Autodesk Inventor part; units mm, degrees
(part 2 of 2)
  spline S97 degree 2 poles (210.6786, 189.7211) (210.6786, 190.1373) (210.1931, 190.6344) (209.8, 190.6344) knots 0 0 0 1 2 2 2
  line L388 (207.8954, 162.25) -> (207.8954, 163.1286)
  line L389 (207.8954, 163.1286) -> (209.589, 169.25)
  line L390 (209.589, 169.25) -> (210.826, 169.25)
  line L391 (210.826, 169.25) -> (209.1555, 163.354)
  line L392 (209.1555, 163.354) -> (210.6526, 163.354)
  line L393 (210.6526, 163.354) -> (210.6526, 164.3829)
  line L394 (210.6526, 164.3829) -> (211.8029, 164.3829)
  line L395 (211.8029, 164.3829) -> (211.8029, 162.25)
  line L396 (211.8029, 162.25) -> (207.8954, 162.25)
  spline S98 degree 2 poles (209.8087, 118.2905) (210.6237, 118.2905) (211.7104, 117.2789) (211.8087, 116.3656) knots 0 0 0 1 2 2 2
  line L397 (211.8087, 116.3656) -> (211.8087, 116.354)
  line L398 (211.8087, 116.354) -> (210.6584, 116.354)
  line L399 (210.6584, 116.354) -> (210.6584, 116.3598)
  spline S99 degree 2 poles (210.6584, 116.3598) (210.6179, 116.7471) (210.1613, 117.1806) (209.7971, 117.1806) knots 0 0 0 1 2 2 2
  spline S100 degree 2 poles (209.7971, 117.1806) (209.3867, 117.1806) (208.9416, 116.6315) (208.9416, 116.1402) knots 0 0 0 1 2 2 2
  line L400 (208.9416, 116.1402) -> (208.9416, 115.5506)
  spline S101 degree 2 poles (208.9416, 115.5506) (208.9416, 115.0535) (209.3636, 114.5159) (209.7624, 114.5159) knots 0 0 0 1 2 2 2
  spline S102 degree 2 poles (209.7624, 114.5159) (210.0283, 114.5159) (210.4618, 114.8049) (210.5948, 115.0708) knots 0 0 0 1 2 2 2
  line L401 (210.5948, 115.0708) -> (211.6584, 115.0708)
  line L402 (211.6584, 115.0708) -> (211.6584, 111.2095)
  line L403 (211.6584, 111.2095) -> (207.9936, 111.2095)
  line L404 (207.9936, 111.2095) -> (207.9936, 112.3136)
  line L405 (207.9936, 112.3136) -> (210.5081, 112.3136)
  line L406 (210.5081, 112.3136) -> (210.5081, 113.7182)
  spline S103 degree 2 poles (210.5081, 113.7182) (210.3347, 113.5679) (209.8491, 113.4061) (209.6121, 113.4061) knots 0 0 0 1 2 2 2
  spline S104 degree 2 poles (209.6121, 113.4061) (208.7451, 113.4061) (207.7913, 114.5275) (207.7913, 115.5506) knots 0 0 0 1 2 2 2
  line L407 (207.7913, 115.5506) -> (207.7913, 116.1402)
  spline S105 degree 2 poles (207.7913, 116.1402) (207.7913, 117.1691) (208.8491, 118.2905) (209.8087, 118.2905) knots 0 0 0 1 2 2 2
  line L408 (212.3467, 92.0147) -> (212.3467, 90.8322)
  line L409 (212.3467, 90.8322) -> (209.7703, 85.25)
  line L410 (209.7703, 85.25) -> (208.3434, 85.25)
  line L411 (208.3434, 85.25) -> (210.8471, 90.7661)
  line L412 (210.8471, 90.7661) -> (207.0948, 90.7661)
  line L413 (207.0948, 90.7661) -> (207.0948, 92.0147)
  line L414 (207.0948, 92.0147) -> (212.3467, 92.0147)
  line L415 (209.004, 93.25) -> (209.004, 88.5398)
  line L416 (209.004, 88.5398) -> (207.7026, 88.5398)
  line L417 (207.7026, 88.5398) -> (207.7026, 93.25)
  line L418 (207.7026, 93.25) -> (209.004, 93.25)
  spline S106 degree 2 poles (209.852, 67.3309) (210.459, 67.3309) (211.4012, 66.8801) (211.9618, 66.0361) (212.0197, 65.435) knots 0 0 0 1 2 3 3 3
  line L419 (212.0197, 65.435) -> (210.8347, 65.435)
  spline S107 degree 2 poles (210.8347, 65.435) (210.7769, 65.828) (210.2971, 66.2211) (209.9214, 66.2211) knots 0 0 0 1 2 2 2
  spline S108 degree 2 poles (209.9214, 66.2211) (209.4879, 66.2211) (209.0197, 65.7471) (209.0197, 65.3194) knots 0 0 0 1 2 2 2
  line L420 (209.0197, 65.3194) -> (209.0197, 65.1286)
  spline S109 degree 2 poles (209.0197, 65.1286) (209.0197, 64.6662) (209.4358, 64.1575) (209.8231, 64.1575) knots 0 0 0 1 2 2 2
  line L421 (209.8231, 64.1575) -> (210.3723, 64.1575)
  line L422 (210.3723, 64.1575) -> (210.3723, 63.0535)
  line L423 (210.3723, 63.0535) -> (209.8231, 63.0535)
  spline S110 degree 2 poles (209.8231, 63.0535) (209.4936, 63.0535) (209.1353, 62.6199) (209.1353, 62.2211) knots 0 0 0 1 2 2 2
  line L424 (209.1353, 62.2211) -> (209.1353, 62.0535)
  spline S111 degree 2 poles (209.1353, 62.0535) (209.1353, 61.6777) (209.5225, 61.2789) (209.8809, 61.2789) knots 0 0 0 1 2 2 2
  spline S112 degree 2 poles (209.8809, 61.2789) (210.1988, 61.2789) (210.6439, 61.6893) (210.7249, 62.1055) knots 0 0 0 1 2 2 2
  line L425 (210.7249, 62.1055) -> (211.904, 62.1055)
  spline S113 degree 2 poles (211.904, 62.1055) (211.7884, 61.1806) (210.6786, 60.1691) (209.852, 60.1691) knots 0 0 0 1 2 2 2
  spline S114 degree 2 poles (209.852, 60.1691) (208.9329, 60.1691) (207.9329, 61.1171) (207.9329, 61.9899) knots 0 0 0 1 2 2 2
  line L426 (207.9329, 61.9899) -> (207.9329, 62.1575)
  spline S115 degree 2 poles (207.9329, 62.1575) (207.9329, 62.6604) (208.4647, 63.4118) (208.9503, 63.591) knots 0 0 0 1 2 2 2
  spline S116 degree 2 poles (208.9503, 63.591) (208.4127, 63.7066) (207.8173, 64.5679) (207.8173, 65.2327) knots 0 0 0 1 2 2 2
  line L427 (207.8173, 65.2327) -> (207.8173, 65.3945)
  spline S117 degree 2 poles (207.8173, 65.3945) (207.8173, 66.3194) (208.8809, 67.3309) (209.852, 67.3309) knots 0 0 0 1 2 2 2
  line L428 (211.7827, 41.7905) -> (211.7827, 40.7673)
  line L429 (211.7827, 40.7673) -> (209.3607, 37.5592)
  spline S118 degree 2 poles (209.3607, 37.5592) (209.1699, 37.3107) (208.9618, 36.7847) (208.9618, 36.5592) knots 0 0 0 1 2 2 2
  line L430 (208.9618, 36.5592) -> (208.9618, 36.5535)
  spline S119 degree 2 poles (208.9618, 36.5535) (208.9618, 36.2009) (209.3954, 35.8136) (209.7884, 35.8136) knots 0 0 0 1 2 2 2
  spline S120 degree 2 poles (209.7884, 35.8136) (210.1584, 35.8136) (210.6324, 36.2818) (210.6844, 36.7095) knots 0 0 0 1 2 2 2
  line L431 (210.6844, 36.7095) -> (210.6844, 36.7153)
  line L432 (210.6844, 36.7153) -> (211.8694, 36.7153)
  line L433 (211.8694, 36.7153) -> (211.8694, 36.7095)
  spline S121 degree 2 poles (211.8694, 36.7095) (211.7653, 35.7558) (210.6671, 34.7095) (209.7942, 34.7095) knots 0 0 0 1 2 2 2
  spline S122 degree 2 poles (209.7942, 34.7095) (208.8289, 34.7095) (207.7769, 35.6633) (207.7769, 36.5361) knots 0 0 0 1 2 2 2
  line L434 (207.7769, 36.5361) -> (207.7769, 36.5419)
  spline S123 degree 2 poles (207.7769, 36.5419) (207.7769, 36.9639) (208.0948, 37.8425) (208.3838, 38.2182) knots 0 0 0 1 2 2 2
  line L435 (208.3838, 38.2182) -> (210.2566, 40.6864)
  line L436 (210.2566, 40.6864) -> (207.7364, 40.6864)
  line L437 (207.7364, 40.6864) -> (207.7364, 41.7905)
  line L438 (207.7364, 41.7905) -> (211.7827, 41.7905)
  line L439 (208.9763, 9.25) -> (208.9763, 16.25)
  line L440 (208.9763, 16.25) -> (210.1266, 16.25)
  line L441 (210.1266, 16.25) -> (210.1266, 10.5564)
  line L442 (210.1266, 10.5564) -> (211.0514, 11.0246)
  line L443 (211.0514, 11.0246) -> (211.0514, 9.8165)
  line L444 (211.0514, 9.8165) -> (210.0341, 9.25)
  line L445 (210.0341, 9.25) -> (208.9763, 9.25)
  line L446 (192.4488, -8.8562) -> (192.4488, -2.7562)
  line L447 (192.4488, -2.7562) -> (193.4512, -2.7562)
  line L448 (193.4512, -2.7562) -> (193.4512, -8.8562)
  line L449 (193.4512, -8.8562) -> (192.4488, -8.8562)
  line L450 (189.0488, -8.8562) -> (189.0488, -2.7562)
  line L451 (189.0488, -2.7562) -> (190.0512, -2.7562)
  line L452 (190.0512, -2.7562) -> (190.0512, -8.8562)
  line L453 (190.0512, -8.8562) -> (189.0488, -8.8562)
  line L454 (189.5777, -6.3225) -> (189.5777, -5.3604)
  line L455 (189.5777, -5.3604) -> (193.0483, -5.3604)
  line L456 (193.0483, -5.3604) -> (193.0483, -6.3225)
  line L457 (193.0483, -6.3225) -> (189.5777, -6.3225)
  line L458 (165.823, -5.5003) -> (167.9386, -5.5003)
  line L459 (167.9386, -5.5003) -> (167.9386, -6.6286)
  spline S124 degree 2 poles (167.9386, -6.6286) (167.9386, -7.3187) (167.3946, -8.3463) (166.4225, -8.9155) (165.7626, -8.9155) knots 0 0 0 1 2 3 3 3
  spline S125 degree 2 poles (165.7626, -8.9155) (165.1027, -8.9155) (164.1104, -8.3815) (163.5614, -7.4144) (163.5614, -6.7646) knots 0 0 0 1 2 3 3 3
  line L460 (163.5614, -6.7646) -> (163.5614, -4.9663)
  spline S126 degree 2 poles (163.5614, -4.9663) (163.5614, -4.2763) (164.1054, -3.2537) (165.0826, -2.6845) (165.7374, -2.6845) knots 0 0 0 1 2 3 3 3
  spline S127 degree 2 poles (165.7374, -2.6845) (166.2764, -2.6845) (167.173, -3.1379) (167.7825, -3.9539) (167.8883, -4.4979) knots 0 0 0 1 2 3 3 3
  line L461 (167.8883, -4.4979) -> (166.8053, -4.4979)
  spline S128 degree 2 poles (166.8053, -4.4979) (166.7045, -4.11) (166.09, -3.697) (165.7374, -3.697) knots 0 0 0 1 2 2 2
  spline S129 degree 2 poles (165.7374, -3.697) (165.2186, -3.697) (164.594, -4.3921) (164.594, -4.9663) knots 0 0 0 1 2 2 2
  line L462 (164.594, -4.9663) -> (164.594, -6.7646)
  spline S130 degree 2 poles (164.594, -6.7646) (164.594, -7.2834) (165.2337, -7.903) (165.7626, -7.903) knots 0 0 0 1 2 2 2
  spline S131 degree 2 poles (165.7626, -7.903) (166.2814, -7.898) (166.906, -7.2381) (166.906, -6.6488) knots 0 0 0 1 2 2 2
  line L463 (166.906, -6.6488) -> (166.906, -6.4624)
  line L464 (166.906, -6.4624) -> (165.823, -6.4624)
  line L465 (165.823, -6.4624) -> (165.823, -5.5003)
  line L466 (138.5626, -8.85) -> (138.5626, -2.75)
  line L467 (138.5626, -2.75) -> (139.5649, -2.75)
  line L468 (139.5649, -2.75) -> (139.5649, -8.85)
  line L469 (139.5649, -8.85) -> (138.5626, -8.85)
  line L470 (138.9806, -3.7121) -> (138.9806, -2.75)
  line L471 (138.9806, -2.75) -> (142.4815, -2.75)
  line L472 (142.4815, -2.75) -> (142.4815, -3.7121)
  line L473 (142.4815, -3.7121) -> (138.9806, -3.7121)
  line L474 (138.9806, -6.3516) -> (138.9806, -5.3895)
  line L475 (138.9806, -5.3895) -> (142.0231, -5.3945)
  line L476 (142.0231, -5.3945) -> (142.0231, -6.3516)
  line L477 (142.0231, -6.3516) -> (138.9806, -6.3516)
  line L478 (112.8963, -8.85) -> (112.8963, -2.75)
  line L479 (112.8963, -2.75) -> (113.8987, -2.75)
  line L480 (113.8987, -2.75) -> (113.8987, -8.85)
  line L481 (113.8987, -8.85) -> (112.8963, -8.85)
  line L482 (113.3094, -3.7121) -> (113.3094, -2.75)
  line L483 (113.3094, -2.75) -> (116.8958, -2.75)
  line L484 (116.8958, -2.75) -> (116.8958, -3.7121)
  line L485 (116.8958, -3.7121) -> (113.3094, -3.7121)
  line L486 (113.3094, -8.85) -> (113.3094, -7.8879)
  line L487 (113.3094, -7.8879) -> (116.8958, -7.8879)
  line L488 (116.8958, -7.8879) -> (116.8958, -8.85)
  line L489 (116.8958, -8.85) -> (113.3094, -8.85)
  line L490 (113.3094, -6.3012) -> (113.3094, -5.3391)
  line L491 (113.3094, -5.3391) -> (116.4374, -5.3441)
  line L492 (116.4374, -5.3441) -> (116.4374, -6.3012)
  line L493 (116.4374, -6.3012) -> (113.3094, -6.3012)
  line L494 (87.7237, -8.85) -> (87.7237, -7.8879)
  line L495 (87.7237, -7.8879) -> (89.1442, -7.8879)
  spline S132 degree 2 poles (89.1442, -7.8879) (89.7638, -7.8879) (90.4488, -7.2633) (90.4488, -6.6991) knots 0 0 0 1 2 2 2
  line L496 (90.4488, -6.6991) -> (90.4488, -4.9009)
  spline S133 degree 2 poles (90.4488, -4.9009) (90.4488, -4.3317) (89.7638, -3.7121) (89.1442, -3.7121) knots 0 0 0 1 2 2 2
  line L497 (89.1442, -3.7121) -> (87.7237, -3.7121)
  line L498 (87.7237, -3.7121) -> (87.7237, -2.75)
  line L499 (87.7237, -2.75) -> (89.119, -2.75)
  spline S134 degree 2 poles (89.119, -2.75) (90.2474, -2.75) (91.4815, -3.8934) (91.4815, -4.9361) knots 0 0 0 1 2 2 2
  line L500 (91.4815, -4.9361) -> (91.4815, -6.6639)
  spline S135 degree 2 poles (91.4815, -6.6639) (91.4815, -7.3338) (90.9374, -8.3161) (89.8847, -8.85) (89.114, -8.85) knots 0 0 0 1 2 3 3 3
  line L501 (89.114, -8.85) -> (87.7237, -8.85)
  line L502 (87.1445, -8.85) -> (87.1445, -2.75)
  line L503 (87.1445, -2.75) -> (88.1469, -2.75)
  line L504 (88.1469, -2.75) -> (88.1469, -8.85)
  line L505 (88.1469, -8.85) -> (87.1445, -8.85)
  spline S136 degree 2 poles (63.8407, -8.9155) (63.1758, -8.9155) (62.2036, -8.3664) (61.6797, -7.3389) (61.6797, -6.6387) knots 0 0 0 1 2 3 3 3
  line L506 (61.6797, -6.6387) -> (61.6797, -4.9663)
  spline S137 degree 2 poles (61.6797, -4.9663) (61.6797, -4.2561) (62.2036, -3.2336) (63.1758, -2.6845) (63.8407, -2.6845) knots 0 0 0 1 2 3 3 3
  spline S138 degree 2 poles (63.8407, -2.6845) (64.3948, -2.6845) (65.2863, -3.158) (65.8757, -4.0345) (65.9865, -4.644) knots 0 0 0 1 2 3 3 3
  line L507 (65.9865, -4.644) -> (64.9539, -4.644)
  spline S139 degree 2 poles (64.9539, -4.644) (64.8783, -4.3417) (64.5509, -3.9136) (64.1026, -3.6768) (63.8407, -3.6768) knots 0 0 0 1 2 3 3 3
  spline S140 degree 2 poles (63.8407, -3.6768) (63.3218, -3.6768) (62.7123, -4.372) (62.7123, -4.9663) knots 0 0 0 1 2 2 2
  line L508 (62.7123, -4.9663) -> (62.7123, -6.6437)
  spline S141 degree 2 poles (62.7123, -6.6437) (62.7123, -7.2331) (63.3218, -7.9232) (63.8407, -7.9232) knots 0 0 0 1 2 2 2
  spline S142 degree 2 poles (63.8407, -7.9232) (64.2336, -7.9232) (64.8481, -7.4245) (64.9539, -6.956) knots 0 0 0 1 2 2 2
  line L509 (64.9539, -6.956) -> (65.9865, -6.956)
  spline S143 degree 2 poles (65.9865, -6.956) (65.8757, -7.5605) (65.2813, -8.442) (64.3948, -8.9155) (63.8407, -8.9155) knots 0 0 0 1 2 3 3 3
  point P0 (0, 0)
  point P1 (0.0104, 102.0099)
  point P2 (1.1, -1.1)
  point P3 (179.6, -1.1)
  point P4 (202.9, -10.5)
  point P5 (-1.1, 1.1)
  point P6 (-10.5, 24.4)
  point P7 (-1.1, 26.6)
  point P8 (-10.5, 49.9)
  point P9 (-1.1, 52.1)
  point P10 (-1.1, 77.6)
  point P11 (-1.1, 154.1)
  point P12 (1.1, 214.5)
  point P13 (24.4, 205.1)
  point P14 (26.6, 214.5)
  point P15 (52.1, 214.5)
  point P16 (214.5, 1.1)
  point P17 (205.1, 24.4)
  point P18 (214.5, 26.6)
  point P19 (205.1, 49.9)
  point P20 (205.1, 75.4)
  point P21 (214.5, 154.1)
  dimension "d0" = 25.5
  dimension "d1" = 25.5
  constraints: 100 coincident, 4 point on line, 2 horizontal, 1 vertical, 72 other
extrude "Extrusion10" cut sketch "Sketch10" against normal blind 0.3 contours S0 | S2 | L198 L199 L200 L201 L202 L208 L207 L206 L203 L205 L204 | L208 L205 L206 L203 | L203 L206 L202 L208 | L202 L206 L207 L208 | L223 L220 L221 L216 L215 L222 L214 L213 L212 L210 L209 | L209 L210 L222 L219 | L222 L210 S4 L211 S5 L212 L214 S6 S7 L215 L217 S8 S9 S10 L218 S11 L219 | L212 L213 L214 L222 | L217 L222 L215 L216 | S12 L224 S13 S14 L225 S15 S16 L226 S17 S18 L227 S19 | L232 L233 L234 L235 L236 L237 L238 L239 L240 | S28 L241 L242 L243 S29 S30 L244 S31 S32 L245 L246 L247 L248 L249 L250 S33 S34 L251 S35 | L252 L253 L254 L255 L256 L259 L258 | L259 L256 L261 L258 | L258 L261 L262 L259 | L261 L256 L257 L258 | L259 L260 L261 L256 | S36 L263 S37 S38 L264 S39 L265 L266 L267 S40 L268 S41 S42 L269 S43 S44 L270 S45 S46 L271 S47 | L272 L273 S48 L274 S49 S50 L275 L276 L277 S51 S52 L278 S53 L279 L280 L281 L282 | L283 L284 L285 L286 L287 L288 L289 | L290 L291 L292 L293 L294 L300 L299 L298 L295 L297 L296 | L300 L297 L298 L295 | L295 L298 L294 L300 | L294 L298 L299 L300 | L315 L312 L313 L308 L307 L314 L306 L305 L304 L302 L301 | L301 L302 L314 L311 | L314 L302 S54 L303 S55 L304 L306 S56 S57 L307 L309 S58 S59 S60 L310 S61 L311 | L304 L305 L306 L314 | L309 L314 L307 L308 | S62 L316 S63 S64 L317 S65 S66 L318 S67 S68 L319 S69 | L331 L328 L329 L324 L323 L330 L321 L320 | L320 L321 L330 L327 | L330 L321 S70 L322 S71 L323 L325 S72 L326 S73 L327 | L323 L324 L325 L330 | L332 L333 L336 L339 L334 L345 L344 L347 L341 L340 L335 | L340 L341 L334 L335 | L333 L334 L339 L336 | L334 L341 L342 L343 | L337 L338 L339 L334 | L347 L344 L345 L334 | L334 L345 L346 L347 | L348 L349 L352 L355 L350 L357 L356 L359 L351 | L349 L350 L355 L352 | L359 L356 L357 L350 | L350 L357 L358 L359 | L353 L354 L355 L350 | L360 L361 S74 S75 L362 S76 S77 L363 S78 S79 L364 S80 S81 L365 L366 L367 | L368 L369 L370 L377 L376 L379 L371 | L379 L376 L377 L370 | L370 L377 L372 L379 | L379 L378 L377 L372 L373 L374 L375 | L372 L377 L378 L379 | S82 L380 S83 S84 L381 S85 S86 L382 S87 S88 L383 S89 | L388 L389 L390 L391 L392 L393 L394 L395 L396 | S98 L397 L398 L399 S99 S100 L400 S101 S102 L401 L402 L403 L404 L405 L406 S103 S104 L407 S105 | L408 L409 L410 L411 L412 L415 L414 | L415 L412 L417 L414 | L414 L417 L418 L415 | L417 L412 L413 L414 | L415 L416 L417 L412 | S106 L419 S107 S108 L420 S109 L421 L422 L423 S110 L424 S111 S112 L425 S113 S114 L426 S115 S116 L427 S117 | L428 L429 S118 L430 S119 S120 L431 L432 L433 S121 S122 L434 S123 L435 L436 L437 L438 | L439 L440 L441 L442 L443 L444 L445 | L446 L457 L456 L455 L447 L448 L449 | L457 L452 L455 L446 | L446 L455 L456 L457 | L457 L454 L455 L452 | L452 L453 L450 L451 L455 L454 L457 | L458 L459 S124 S125 L460 S126 S127 L461 S128 S129 L462 S130 S131 L463 L464 L465 | L466 L467 L470 L473 L468 L475 L474 L477 L469 | L467 L468 L473 L470 | L477 L474 L475 L468 | L468 L475 L476 L477 | L471 L472 L473 L468 | L478 L479 L482 L485 L480 L491 L490 L493 L487 L486 L481 | L486 L487 L480 L481 | L479 L480 L485 L482 | L480 L487 L488 L489 | L483 L484 L485 L480 | L493 L490 L491 L480 | L480 L491 L492 L493 | L505 L502 L503 L498 L497 L504 L495 L494 | L494 L495 L504 L501 | L504 L495 S132 L496 S133 L497 L499 S134 L500 S135 L501 | L497 L498 L499 L504 | S136 L506 S137 S138 L507 S139 S140 L508 S141 S142 L509 S143
sketch "Sketch11" plane through (0, 2.8, 0) normal (0, 1, 0) x (1, 0, 0)
  circle A0 centre (12.75, 191.25) radius 3 projected
  circle A1 centre (38.25, 191.25) radius 3 projected
  circle A2 centre (63.75, 191.25) radius 3 projected
  circle A3 centre (89.25, 191.25) radius 3 projected
  circle A4 centre (114.75, 191.25) radius 3 projected
  circle A5 centre (140.25, 191.25) radius 3 projected
  circle A6 centre (165.75, 191.25) radius 3 projected
  circle A7 centre (191.25, 191.25) radius 3 projected
  circle A8 centre (191.25, 165.75) radius 3 projected
  circle A9 centre (165.75, 165.75) radius 3 projected
  circle A10 centre (114.75, 165.75) radius 3 projected
  circle A11 centre (63.75, 165.75) radius 3 projected
  circle A12 centre (89.25, 140.25) radius 3 projected
  circle A13 centre (89.25, 165.75) radius 3 projected
  circle A14 centre (38.25, 165.75) radius 3 projected
  circle A15 centre (12.75, 165.75) radius 3 projected
  circle A16 centre (140.25, 165.75) radius 3 projected
  circle A17 centre (191.25, 140.25) radius 3 projected
  circle A18 centre (165.75, 140.25) radius 3 projected
  circle A19 centre (140.25, 140.25) radius 3 projected
  circle A20 centre (114.75, 140.25) radius 3 projected
  circle A21 centre (114.75, 114.75) radius 3 projected
  circle A22 centre (165.75, 114.75) radius 3 projected
  circle A23 centre (140.25, 89.25) radius 3 projected
  circle A24 centre (140.25, 114.75) radius 3 projected
  circle A25 centre (191.25, 114.75) radius 3 projected
  circle A26 centre (89.25, 114.75) radius 3 projected
  circle A27 centre (63.75, 114.75) radius 3 projected
  circle A28 centre (38.25, 114.75) radius 3 projected
  circle A29 centre (12.75, 114.75) radius 3 projected
  circle A30 centre (38.25, 89.25) radius 3 projected
  circle A31 centre (12.75, 89.25) radius 3 projected
  circle A32 centre (63.75, 89.25) radius 3 projected
  circle A33 centre (89.25, 89.25) radius 3 projected
  circle A34 centre (63.75, 140.25) radius 3 projected
  circle A35 centre (38.25, 140.25) radius 3 projected
  circle A36 centre (12.75, 140.25) radius 3 projected
  circle A37 centre (114.75, 89.25) radius 3 projected
  circle A38 centre (165.75, 89.25) radius 3 projected
  circle A39 centre (191.25, 89.25) radius 3 projected
  circle A40 centre (191.25, 63.75) radius 3 projected
  circle A41 centre (165.75, 63.75) radius 3 projected
  circle A42 centre (89.25, 63.75) radius 3 projected
  circle A43 centre (140.25, 63.75) radius 3 projected
  circle A44 centre (114.75, 63.75) radius 3 projected
  circle A45 centre (63.75, 63.75) radius 3 projected
  circle A46 centre (38.25, 63.75) radius 3 projected
  circle A47 centre (12.75, 63.75) radius 3 projected
  circle A48 centre (191.25, 38.25) radius 3 projected
  circle A49 centre (165.75, 38.25) radius 3 projected
  circle A50 centre (140.25, 38.25) radius 3 projected
  circle A51 centre (114.75, 38.25) radius 3 projected
  circle A52 centre (89.25, 38.25) radius 3 projected
  circle A53 centre (63.75, 38.25) radius 3 projected
  circle A54 centre (38.25, 38.25) radius 3 projected
  circle A55 centre (12.75, 38.25) radius 3 projected
  circle A56 centre (12.75, 12.75) radius 3 projected
  circle A57 centre (38.25, 12.75) radius 3 projected
  circle A58 centre (63.75, 12.75) radius 3 projected
  circle A59 centre (89.25, 12.75) radius 3 projected
  circle A60 centre (114.75, 12.75) radius 3 projected
  circle A61 centre (140.25, 12.75) radius 3 projected
  circle A62 centre (165.75, 12.75) radius 3 projected
  circle A63 centre (191.25, 12.75) radius 3 projected
  circle A64 centre (5.5, 198.5) radius 1.75
  circle A65 centre (20, 184) radius 1.75
  line L0 (1.5, 202.5) -> (24, 202.5) projected
  line L1 (1.5, 180) -> (1.5, 202.5) projected
  line L2 (24, 180) -> (1.5, 180) projected
  line L3 (24, 202.5) -> (24, 180) projected
  circle A66 centre (31, 198.5) radius 1.75
  circle A67 centre (45.5, 184) radius 1.75
  circle A68 centre (56.5, 198.5) radius 1.75
  circle A69 centre (71, 184) radius 1.75
  circle A70 centre (82, 198.5) radius 1.75
  circle A71 centre (96.5, 184) radius 1.75
  circle A72 centre (107.5, 198.5) radius 1.75
  circle A73 centre (122, 184) radius 1.75
  circle A74 centre (133, 198.5) radius 1.75
  circle A75 centre (147.5, 184) radius 1.75
  circle A76 centre (158.5, 198.5) radius 1.75
  circle A77 centre (173, 184) radius 1.75
  circle A78 centre (184, 198.5) radius 1.75
  circle A79 centre (198.5, 184) radius 1.75
  circle A80 centre (5.5, 173) radius 1.75
  circle A81 centre (20, 158.5) radius 1.75
  circle A82 centre (31, 173) radius 1.75
  circle A83 centre (45.5, 158.5) radius 1.75
  circle A84 centre (56.5, 173) radius 1.75
  circle A85 centre (71, 158.5) radius 1.75
  circle A86 centre (82, 173) radius 1.75
  circle A87 centre (96.5, 158.5) radius 1.75
  circle A88 centre (107.5, 173) radius 1.75
  circle A89 centre (122, 158.5) radius 1.75
  circle A90 centre (133, 173) radius 1.75
  circle A91 centre (147.5, 158.5) radius 1.75
  circle A92 centre (158.5, 173) radius 1.75
  circle A93 centre (173, 158.5) radius 1.75
  circle A94 centre (184, 173) radius 1.75
  circle A95 centre (198.5, 158.5) radius 1.75
  circle A96 centre (5.5, 147.5) radius 1.75
  circle A97 centre (20, 133) radius 1.75
  circle A98 centre (31, 147.5) radius 1.75
  circle A99 centre (45.5, 133) radius 1.75
  circle A100 centre (56.5, 147.5) radius 1.75
  circle A101 centre (71, 133) radius 1.75
  circle A102 centre (82, 147.5) radius 1.75
  circle A103 centre (96.5, 133) radius 1.75
  circle A104 centre (107.5, 147.5) radius 1.75
  circle A105 centre (122, 133) radius 1.75
  circle A106 centre (133, 147.5) radius 1.75
  circle A107 centre (147.5, 133) radius 1.75
  circle A108 centre (158.5, 147.5) radius 1.75
  circle A109 centre (173, 133) radius 1.75
  circle A110 centre (184, 147.5) radius 1.75
  circle A111 centre (198.5, 133) radius 1.75
  circle A112 centre (5.5, 122) radius 1.75
  circle A113 centre (20, 107.5) radius 1.75
  circle A114 centre (31, 122) radius 1.75
  circle A115 centre (45.5, 107.5) radius 1.75
  circle A116 centre (56.5, 122) radius 1.75
  circle A117 centre (71, 107.5) radius 1.75
  circle A118 centre (82, 122) radius 1.75
  circle A119 centre (96.5, 107.5) radius 1.75
  circle A120 centre (107.5, 122) radius 1.75
  circle A121 centre (122, 107.5) radius 1.75
  circle A122 centre (133, 122) radius 1.75
  circle A123 centre (147.5, 107.5) radius 1.75
  circle A124 centre (158.5, 122) radius 1.75
  circle A125 centre (173, 107.5) radius 1.75
  circle A126 centre (184, 122) radius 1.75
  circle A127 centre (198.5, 107.5) radius 1.75
  circle A128 centre (5.5, 96.5) radius 1.75
  circle A129 centre (20, 82) radius 1.75
  circle A130 centre (31, 96.5) radius 1.75
  circle A131 centre (45.5, 82) radius 1.75
  circle A132 centre (56.5, 96.5) radius 1.75
  circle A133 centre (71, 82) radius 1.75
  circle A134 centre (82, 96.5) radius 1.75
  circle A135 centre (96.5, 82) radius 1.75
  circle A136 centre (107.5, 96.5) radius 1.75
  circle A137 centre (122, 82) radius 1.75
  circle A138 centre (133, 96.5) radius 1.75
  circle A139 centre (147.5, 82) radius 1.75
  circle A140 centre (158.5, 96.5) radius 1.75
  circle A141 centre (173, 82) radius 1.75
  circle A142 centre (184, 96.5) radius 1.75
  circle A143 centre (198.5, 82) radius 1.75
  circle A144 centre (5.5, 71) radius 1.75
  circle A145 centre (20, 56.5) radius 1.75
  circle A146 centre (31, 71) radius 1.75
  circle A147 centre (45.5, 56.5) radius 1.75
  circle A148 centre (56.5, 71) radius 1.75
  circle A149 centre (71, 56.5) radius 1.75
  circle A150 centre (82, 71) radius 1.75
  circle A151 centre (96.5, 56.5) radius 1.75
  circle A152 centre (107.5, 71) radius 1.75
  circle A153 centre (122, 56.5) radius 1.75
  circle A154 centre (133, 71) radius 1.75
  circle A155 centre (147.5, 56.5) radius 1.75
  circle A156 centre (158.5, 71) radius 1.75
  circle A157 centre (173, 56.5) radius 1.75
  circle A158 centre (184, 71) radius 1.75
  circle A159 centre (198.5, 56.5) radius 1.75
  circle A160 centre (5.5, 45.5) radius 1.75
  circle A161 centre (20, 31) radius 1.75
  circle A162 centre (31, 45.5) radius 1.75
  circle A163 centre (45.5, 31) radius 1.75
  circle A164 centre (56.5, 45.5) radius 1.75
  circle A165 centre (71, 31) radius 1.75
  circle A166 centre (82, 45.5) radius 1.75
  circle A167 centre (96.5, 31) radius 1.75
  circle A168 centre (107.5, 45.5) radius 1.75
  circle A169 centre (122, 31) radius 1.75
  circle A170 centre (133, 45.5) radius 1.75
  circle A171 centre (147.5, 31) radius 1.75
  circle A172 centre (158.5, 45.5) radius 1.75
  circle A173 centre (173, 31) radius 1.75
  circle A174 centre (184, 45.5) radius 1.75
  circle A175 centre (198.5, 31) radius 1.75
  circle A176 centre (5.5, 20) radius 1.75
  circle A177 centre (20, 5.5) radius 1.75
  circle A178 centre (31, 20) radius 1.75
  circle A179 centre (45.5, 5.5) radius 1.75
  circle A180 centre (56.5, 20) radius 1.75
  circle A181 centre (71, 5.5) radius 1.75
  circle A182 centre (82, 20) radius 1.75
  circle A183 centre (96.5, 5.5) radius 1.75
  circle A184 centre (107.5, 20) radius 1.75
  circle A185 centre (122, 5.5) radius 1.75
  circle A186 centre (133, 20) radius 1.75
  circle A187 centre (147.5, 5.5) radius 1.75
  circle A188 centre (158.5, 20) radius 1.75
  circle A189 centre (173, 5.5) radius 1.75
  circle A190 centre (184, 20) radius 1.75
  circle A191 centre (198.5, 5.5) radius 1.75
  line L4 (202.5, 24) -> (202.5, 1.5) projected
  line L5 (202.5, 1.5) -> (180, 1.5) projected
  point P0 (0, 0)
  dimension "d59" = 3.5
  dimension "d60" = 4
  dimension "d61" = 4
  dimension "d62" = 4
  dimension "d63" = 4
  dimension "d66" = 25.5
  dimension "d69" = 25.5
  dimension "d72" = 4
  dimension "d73" = 4
  constraints: 128 centre point, 1 equal radius, 1 horizontal, 1 vertical, 252 other
  measures "d59" diameter of A64
  measures "d60" distance from line of L0 A64.centre
  measures "d61" distance from line of L1 A64.centre
  measures "d62" distance from line of L2 A65.centre
  measures "d63" distance from line of L3 A65.centre
  measures "d66" distance of A64.centre A66.centre
  measures "d69" distance of A64.centre A80.centre
  measures "d72" distance from line of A191.centre L4
  measures "d73" distance from line of L5 A191.centre
extrude "Extrusion11" cut sketch "Sketch11" against normal blind 1.5 contours A0 | A1 | A2 | A3 | A4 | A5 | A6 | A7 | A8 | A9 | A10 | A11 | A12 | A13 | A14 | A15 | A16 | A17 | A18 | A19 | A20 | A21 | A22 | A23 | A24 | A25 | A26 | A27 | A28 | A29 | A30 | A31 | A32 | A33 | A34 | A35 | A36 | A37 | A38 | A39 | A40 | A41 | A42 | A43 | A44 | A45 | A46 | A47 | A48 | A49 | A50 | A51 | A52 | A53 | A54 | A55 | A56 | A57 | A58 | A59 | A60 | A61 | A62 | A63 | A64 | A65 | A66 | A67 | A68 | A69 | A70 | A71 | A72 | A73 | A74 | A75 | A76 | A77 | A78 | A79 | A80 | A81 | A82 | A83 | A84 | A85 | A86 | A87 | A88 | A89 | A90 | A91 | A92 | A93 | A94 | A95 | A96 | A97 | A98 | A99 | A100 | A101 | A102 | A103 | A104 | A105 | A106 | A107 | A108 | A109 | A110 | A111 | A112 | A113 | A114 | A115 | A116 | A117 | A118 | A119 | A120 | A121 | A122 | A123 | A124 | A125 | A126 | A127 | A128 | A129 | A130 | A131 | A132 | A133 | A134 | A135 | A136 | A137 | A138 | A139 | A140 | A141 | A142 | A143 | A144 | A145 | A146 | A147 | A148 | A149 | A150 | A151 | A152 | A153 | A154 | A155 | A156 | A157 | A158 | A159 | A160 | A161 | A162 | A163 | A164 | A165 | A166 | A167 | A168 | A169 | A170 | A171 | A172 | A173 | A174 | A175 | A176 | A177 | A178 | A179 | A180 | A181 | A182 | A183 | A184 | A185 | A186 | A187 | A188 | A189 | A190 | A191
sketch "Sketch12" plane through (0, 2.8, 0) normal (0, 1, 0) x (1, 0, 0)
  circle A0 centre (5.5, 20) radius 1.75 projected
  circle A1 centre (20, 5.5) radius 1.75 projected
  circle A2 centre (12.75, 12.75) radius 3 projected
  line L0 (1.5, 24) -> (24, 24) projected
  line L1 (1.5, 1.5) -> (1.5, 24) projected
  line L2 (24, 1.5) -> (1.5, 1.5) projected
  line L3 (24, 24) -> (24, 1.5) projected
  point P0 (0, 0)
extrude "Extrusion12" add sketch "Sketch12" along normal blind 0.4 separate body contours A0 | A1 | A2 | L0 L3 L2 L1
chamfer "Chamfer5" distance 0.4 angle 45 4 edges at (1.5, 3.2, -12.75) (12.75, 3.2, -1.5) (24, 3.2, -12.75) (12.75, 3.2, -24)
sketch "Sketch13" plane through (0, 2.8, 0) normal (0, -1, 0) x (1, 0, 0)
  circle A0 centre (5.5, -20) radius 1.75 projected
  circle A1 centre (20, -5.5) radius 1.75 projected
  circle A2 centre (12.75, -12.75) radius 3 projected
  circle A3 centre (5.5, -20) radius 1.55
  circle A4 centre (20, -5.5) radius 1.55
  point P0 (0, 0)
  dimension "d81" = 0.2
  dimension "d82" = 0.2
  constraints: 2 centre point
  measures "d81" radial gap between concentric circles of A0 A3
  measures "d82" radial gap between concentric circles of A1 A4
extrude "Extrusion13" add sketch "Sketch13" along normal blind 1.2 contours A3 | A4 bodies 2
chamfer "Chamfer6" distance 0.4 angle 45 2 edges at (3.95, 1.6, -20) (18.45, 1.6, -5.5)
equation "\"d9\" = 0.5 * d8"
equation "\"d11\" = 0.5 * d10"
